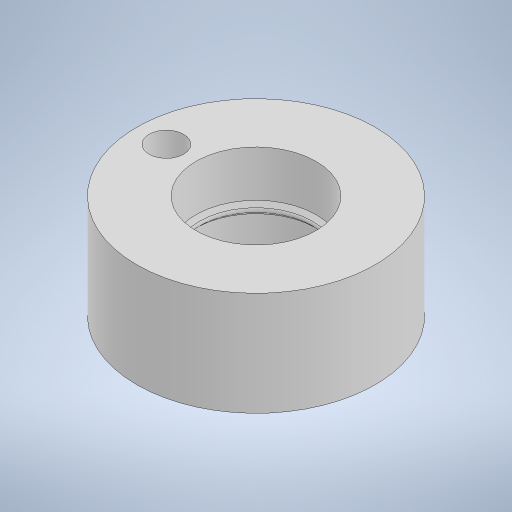
# Autodesk Inventor part: Spool
Saved by Autodesk Inventor 2023.4 (Build 274418000, 418)
## iProperties
Created: 2024-05-13
Part Number: Spool
Material: Generic
Document SubType Name: Modeling
Designer: Nathan Cai
Density: 1 g/cm^3
Appearance: Default
Author: Nathan Cai
Autodesk Inventor part; units mm, degrees
ref_plane "YZ Plane" through (0, 0, 0) normal (1, 0, 0) x (0, 1, 0)
ref_plane "XZ Plane" through (0, 0, 0) normal (0, 1, 0) x (-1, 0, 0)
ref_plane "XY Plane" through (0, 0, 0) normal (0, 0, 1) x (1, 0, 0)
sketch "Sketch1" plane through (0, 0, 0) normal (1, 0, 0) x (0, 1, 0)
  line L0 (0, 0) -> (9, 0)
  line L1 (9, 0) -> (9, -10.3188)
  line L2 (9, -10.3188) -> (0, -10.3188)
  line L3 (0, -10.3188) -> (0, 0)
  line L4 (9, 0) -> (0, 0)
  line L5 (0, 0) -> (0, -5.2)
  line L6 (0, -5.2) -> (9, -5.2)
  line L7 (9, -5.2) -> (9, 0)
  line L8 (5, -5.2) -> (4, -5.2)
  line L9 (4, -5.2) -> (4, -4.7)
  line L10 (4, -4.7) -> (5, -4.7)
  line L11 (5, -4.7) -> (5, -5.2)
  dimension "d0" = 9
  dimension "d1" = 5.2
  dimension "d2" = 10.3187
  dimension "d3" = 0.5
  dimension "d4" = 4
  dimension "d5" = 4
  constraints: 24 end point, 6 parallel, 3 horizontal, 3 perpendicular, 2 point on line
  measures "d0" distance of L1.end L2.end
  measures "d1" distance of L5.end L4.end
  measures "d2" distance between parallel lines of L0 L2
  measures "d3" distance of L8.end L9.end
  measures "d4" distance between parallel lines of L3 L9
  measures "d5" distance between parallel lines of L1 L11
revolve "Revolution1" add sketch "Sketch1" angle 360 about axis through (0, 0, 0) along (0, 1, 0) contours L6 L1 L2 L3 | L9 L10 L11 L6
chamfer "Chamfer1" distance 0.5 angle 45 2 edges at (0, 4, 4.7) (0, 5, 4.7)
fillet "Fillet1" radius 0.25 2 edges at (0, 4.4999, 4.7) (0, 4.5001, 4.7)
sketch "Sketch2" plane through (0, 9, 0) normal (0, 1, 0) x (1, 0, 0)
  circle A0 centre (0, 0) radius 5.2 projected
  line L0 (-5.2, 0) -> (-10.3188, 0) construction
  circle A1 centre (-7.7594, 0) radius 1.5
  circle A2 centre (0, 0) radius 10.3188 projected
  dimension "d11" = 3
  constraints: 2 end point, 2 horizontal alignment, 1 centre point, 1 horizontal, 1 midpoint, 1 point on line, 2 other
  measures "d11" diameter of A1
extrude "Extrusion1" cut sketch "Sketch2" against normal through all contours A1
equation "\"d5\" = d4"
body "Solid1"
